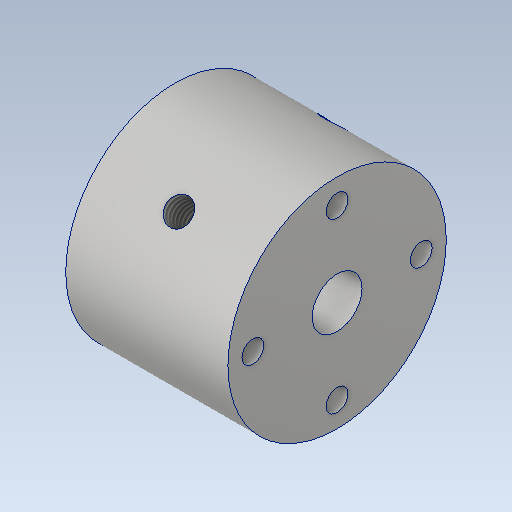
# Autodesk Inventor part: piasta_kola_napedowego_fi8
Saved by Autodesk Inventor 2020 (Build 240168000, 168)
## iProperties
Created: 2019-05-26
Part Number: piasta_kola_napedowego_fi8
Material: Aluminum 6061
Document SubType Name: Modeling
Designer: Besiu
Density: 2.7 g/cm^3
Appearance: Aluminum - Flat
Mass: 60.323 g
Surface Area: 67.0384 cm^2
Volume: 22.3418 cm^3
Author: Besiu
Autodesk Inventor part; units mm, degrees
note: some values were not read from the file. Chosen so that the rebuilt part matches the saved one: direction of "Otwór5"; direction of "Otwór6".
ref_plane "YZ Plane" through (0, 0, 0) normal (1, 0, 0) x (0, 1, 0)
sketch "Szkic1" plane through (0, 0, 0) normal (1, 0, 0) x (0, 1, 0)
  circle A0 centre (0, 0) radius 17.5
  dimension "d0" = 35
  constraints: 1 centre point, 1 coincident
  measures "d0" diameter of A0
extrude "Wyciągnięcie proste1" add sketch "Szkic1" along normal blind 26
sketch "Szkic2" plane through (26, 0, 0) normal (1, 0, 0) x (0, 0, -1)
  point P0 (0, 0)
  point P1 (0, 0)
  constraints: 1 coincident
hole "Otwór1" at (26, 0, 0) direction (-1, 0, 0) diameter 8 end through all
sketch "Szkic3" plane through (26, 0, 0) normal (1, 0, 0) x (0, 0, -1)
  point P0 (0, 0)
  point P1 (13.5, 0)
  point P2 (0, 13.5)
  point P3 (-13.5, 0)
  point P4 (0, -13.5)
  dimension "d10" = 13.5
  dimension "d13" = 360
  constraints: 1 horizontal alignment, 5 other
  measures "d10" distance of point (13.5, 0) point (0, 0)
hole "Otwór2" at (26, 0, -13.5) at (26, 13.5, 0) at (26, 0, 13.5) at (26, -13.5, 0) direction (-1, 0, 0) diameter 3.5 depth 26 tip angle 118
sketch "Szkic4" plane through (26, 0, 0) normal (1, 0, 0) x (0, 0, -1)
  line L0 (0, 0) -> (-12.3744, 12.3744)
  line L1 (0, 0) -> (17.5, 0) construction
  line L2 (0, 0) -> (12.3744, 12.3744)
  line L3 (0, 0) -> (17.5, 0) construction
  dimension "d22" = 17.5
  dimension "d23" = 135
  dimension "d24" = 17.5
  dimension "d25" = 45
  constraints: 8 end point, 2 equal length, 2 horizontal
  measures "d22" distance of L0.start L0.end
  measures "d23" angle of L1 L0
  measures "d24" distance of L0.start L2.end
  measures "d25" angle of L3 L2
ref_plane "Płaszczyzna konstrukcyjna1" through (26, 12.3744, 12.3744) normal (0, 0.7071068, 0.7071068) x (-1, 0, 0)
ref_plane "Płaszczyzna konstrukcyjna2" through (26, 12.3744, -12.3744) normal (0, 0.7071068, -0.7071068) x (-1, 0, 0)
sketch "Szkic10" plane through (26, 12.3744, 12.3744) normal (0, 0.7071068, 0.7071068) x (-1, 0, 0)
  line L0 (26, -17.5) -> (26, 17.5) projected
  line L1 (0, 17.5) -> (0, -17.5) projected
  line L2 (26, 17.5) -> (0, 17.5) projected
  line L3 (26, -17.5) -> (0, -17.5) projected
  point P0 (26, 0)
  point P1 (13, 0)
  dimension "d54" = 13
  dimension "d55" = 26
  dimension "d56" = 35
  dimension "d57" = 17.5
  measures "d54" distance from line of L0 point (13, 0)
  measures "d55" distance between parallel lines of L1 L0
  measures "d56" distance between parallel lines of L2 L3
  measures "d57" distance from line of L3 point (13, 0)
hole "Otwór5" at (13, 12.3744, 12.3744) direction (0, -0.7071068, -0.7071068) diameter 4.134 end up to surface thread size "M5x0.8" class "6H" standard "ANSI Metric M Profile"
sketch "Szkic12" plane through (26, 12.3744, -12.3744) normal (0, 0.7071068, -0.7071068) x (-1, 0, 0)
  line L0 (26, 17.5) -> (0, 17.5) projected
  line L1 (26, -17.5) -> (26, 17.5) projected
  line L2 (26, -17.5) -> (0, -17.5) projected
  line L3 (0, 17.5) -> (0, -17.5) projected
  point P0 (26, 0)
  point P1 (13, 0)
  dimension "d67" = 35
  dimension "d68" = 26
  dimension "d69" = 13
  dimension "d70" = 17.5
  measures "d67" distance between parallel lines of L2 L0
  measures "d68" distance between parallel lines of L3 L1
  measures "d69" distance from line of L1 point (13, 0)
  measures "d70" distance from line of L2 point (13, 0)
hole "Otwór6" at (13, 12.3744, -12.3744) direction (0, -0.7071068, 0.7071068) diameter 4.134 end up to surface thread size "M5x0.8" class "6H" standard "ANSI Metric M Profile"
equation "\"d0\" = radius"
equation "\"d16\" = d1"
equation "\"d20\" = d1"
equation "\"d22\" = 0.5 * radius"
equation "\"d24\" = d22"
equation "\"d54\" = 0.5 * d55"
equation "\"d57\" = 0.5 * d56"
equation "\"d69\" = 0.5 * d68"
equation "\"d70\" = 0.5 * d67"
equation "\"radius\" = 35"
equation "\"d1\" = 26"
